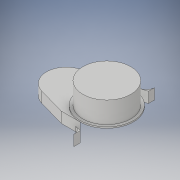
# Autodesk Inventor part: new_cigueñal
Saved by Autodesk Inventor 2019.3 (Build 233278000, 278)
## iProperties
Created: 2019-06-27
Part Number: new_cigueñal
Material: Generic
Document SubType Name: Modeling
Designer: Usuario
Density: 1 g/cm^3
Appearance: Default
Author: Usuario
Autodesk Inventor part; units mm, degrees
ref_plane "YZ Plane" through (0, 0, 0) normal (1, 0, 0) x (0, 1, 0)
ref_plane "XZ Plane" through (0, 0, 0) normal (0, 1, 0) x (-1, 0, 0)
ref_plane "XY Plane" through (0, 0, 0) normal (0, 0, 1) x (1, 0, 0)
sketch "Sketch2" plane through (0, 0, 0) normal (0, 1, 0) x (-1, 0, 0)
  circle A0 centre (0, 0) radius 28.575
  dimension "d0" = 57.15
  constraints: 1 centre point, 1 coincident
  measures "d0" diameter of A0
extrude "Extrusion1" add sketch "Sketch2" against normal blind 25.4
sketch "Sketch3" plane through (0, -25.4, 0) normal (0, -1, 0) x (1, 0, 0)
  circle A0 centre (0, 0) radius 31.75
  dimension "d3" = 63.5
  constraints: 1 centre point, 1 coincident
  measures "d3" diameter of A0
extrude "Extrusion2" add sketch "Sketch3" along normal blind 1.5875
sketch "Sketch4" plane through (0, -26.9875, 0) normal (0, -1, 0) x (1, 0, 0)
  arc A0 (8.89, -56.9095) -> (8.89, 57.3905) centre (8.89, 0.2405) ccw
  arc A1 (-54.665, 22.7287) -> (-54.665, -22.7287) centre (-48.2595, 0) ccw
  line L0 (8.89, -56.9095) -> (8.89, 57.3905) construction
  line L1 (8.89, -40.64) -> (-54.665, -22.7287)
  line L2 (0, 0) -> (66.0395, 0) construction
  line L3 (8.89, 40.64) -> (-54.665, 22.7287)
  line L4 (8.89, 40.64) -> (8.89, 57.3905)
  line L5 (8.89, -40.64) -> (8.89, -56.9095)
  circle A2 centre (0, 0) radius 28.575
  line L6 (18.7922, 40.64) -> (8.89, 40.64)
  line L7 (8.89, -40.64) -> (18.7922, -40.64)
  arc A3 (18.7922, -40.64) -> (18.7922, 40.64) centre (0.7869, 0) ccw
  line L8 (18.7922, 40.64) -> (18.7922, 56.5261)
  line L9 (18.7922, -56.045) -> (18.7922, -40.64)
  line L10 (18.7922, -21.5263) -> (18.7922, 21.5263)
  point P0 (-61.1412, -20.9035)
  point P1 (38.37, -48.7192)
  point P2 (-61.1412, 20.9035)
  dimension "d6" = 114.3
  dimension "d7" = 47.2281
  dimension "d8" = 57.15
  dimension "d11" = 81.28
  dimension "d30" = 44.45
  constraints: 22 end point, 12 point on circle, 4 centre point, 3 perpendicular, 2 symmetric about line, 2 tangent, 1 coincident, 1 collinear, 1 horizontal, 1 parallel, 1 point on line, 1 vertical
  measures "d6" diameter of A0
  measures "d7" diameter of A1
  measures "d8" distance of A1.centre A0.centre
  measures "d11" distance of L3.start L1.start
  measures "d30" radius of A3
extrude "Extrusion3" add sketch "Sketch4" along normal blind 12.7 contours L5 L7 L9 A0 | L9 A3 L8 A0 | L1 A1 L3 L6 A3 L7 | L8 L6 L4 A0 | A2 L10 | L10 A2
fillet "Fillet1" radius 9.906 1 edges at (8.89, -33.3375, 40.64)
fillet "Fillet2" radius 9.906 1 edges at (8.89, -33.3375, -40.64)
sketch "Sketch10" plane through (0, -26.9875, 0) normal (0, 1, 0) x (1, 0, 0)
  circle A0 centre (0, 0) radius 31.75 projected
  line L0 (0, -31.75) -> (-22.6545, -31.75)
  line L1 (1.6711, -38.6055) -> (-54.665, -22.7287) construction
  line L2 (0, -38.1346) -> (-54.665, -22.7287) construction
  line L3 (0, 31.75) -> (-22.6545, 31.75)
  line L4 (-54.665, 22.7287) -> (1.6711, 38.6055) construction
  line L5 (0, 38.1346) -> (-51.396, 23.65) construction
  line L6 (-22.6545, 31.75) -> (8.89, 40.64)
  arc A1 (8.89, -57.3905) -> (8.89, 56.9095) centre (8.89, -0.2405) ccw projected
  line L7 (8.89, 56.9095) -> (8.89, 40.64)
  line L8 (8.89, 40.64) -> (-22.6545, 31.75)
  line L9 (0, -31.75) -> (-22.6545, -31.75)
  line L10 (8.89, -40.64) -> (-22.6545, -31.75)
  line L11 (8.89, -57.3905) -> (8.89, -40.64)
  line L12 (8.89, 48.1401) -> (8.89, 56.9095) projected
  arc A2 (8.89, -57.3905) -> (8.89, 56.9095) centre (8.89, -0.2405) ccw
  arc A3 (0, -31.75) -> (0, 31.75) centre (0, 0) ccw
  point P0 (0, 0)
  constraints: 20 end point, 6 point on circle, 5 point on line, 5 tangent, 4 collinear, 2 centre point, 2 horizontal, 1 perpendicular, 1 vertical
extrude "Extrusion9" cut sketch "Sketch10" against normal blind 25.4
body "Solid1"
